Autodesk Fusion 360 part; units mm, degrees
note: some values were not read from the file. Chosen so that the rebuilt part matches the saved one: which bodies a step acts on; which face or edge a step refers to. Set by a fixed rule: which sketch regions a step uses.
(part 2 of 2)
  constraint coincident L37.end L318
  constraint collinear L368 L379
  constraint vertical L402
  constraint vertical L419
  constraint vertical L410
  constraint vertical L381
  constraint midpoint P2 L306
  constraint horizontal L424
  constraint vertical L427
  constraint vertical L414
  constraint horizontal L442
  constraint vertical L328
  constraint horizontal L440
  constraint horizontal L417
  constraint coincident L38.end L318
  constraint coincident L39.start L318
  constraint coincident L46.end L318
  constraint coincident L45.start L318
  constraint coincident L43.end L318
  constraint coincident L44.start L318
  constraint coincident L49.end L318
  constraint coincident L47.start L318
  constraint collinear L368 L424
  constraint collinear L424 L442
  constraint collinear L440 L442
  constraint collinear L417 L440
  constraint horizontal L421
  constraint vertical L413
  constraint vertical L395
  constraint horizontal L412
  constraint vertical L401
  constraint horizontal L429
  constraint horizontal L439
  constraint collinear L412 L421
  constraint collinear L412 L429
  constraint collinear L429 L439
  constraint horizontal L420
  constraint vertical L390
  constraint vertical L433
  constraint horizontal L358
  constraint vertical L378
  constraint collinear L358 L420
  constraint equal L368 L424
  constraint equal L424 L442
  constraint equal L440 L442
  constraint equal L417 L440
  constraint equal L417 L421
  constraint equal L412 L421
  constraint equal L412 L429
  constraint equal L429 L439
  constraint equal L420 L439
  constraint equal L358 L420
  constraint coincident L63.start L318
  constraint coincident L64.end L318
  constraint coincident L65.start L318
  constraint coincident L67.end L318
  constraint coincident L50.start L318
  constraint coincident L57.end L318
  constraint coincident L59.start L318
  constraint coincident L60.end L318
  constraint coincident L52.start L318
  constraint coincident L53.end L318
  constraint coincident L54.start L318
  constraint collinear L420 L439
  constraint collinear L417 L421
  constraint vertical L369
  constraint vertical L391
  constraint vertical L370
  constraint coincident L107.end L333
  constraint perpendicular L333 L356
  constraint coincident L80.start L333
  constraint perpendicular L333 L403
  constraint coincident L120.end L333
  constraint perpendicular L333 L343
  constraint collinear L303 L377
  constraint coincident L108.start L333
  constraint perpendicular L333 L371
  constraint perpendicular L330 L371
  constraint coincident L113.end L333
  constraint perpendicular L333 L351
  constraint coincident L119.start L333
  constraint perpendicular L333 L389
  constraint perpendicular L351 L375
  constraint coincident L86.end L333
  constraint perpendicular L333 L397
  constraint coincident L98.start L333
  constraint perpendicular L333 L380
  constraint perpendicular L351 L441
  constraint coincident L103.end L333
  constraint perpendicular L333 L382
  constraint coincident L128.start L333
  constraint perpendicular L333 L434
  constraint perpendicular L351 L405
  constraint coincident L130.end L333
  constraint perpendicular L333 L388
  constraint coincident L126.start L333
  constraint perpendicular L333 L357
  constraint perpendicular L351 L374
  constraint coincident L129.end L333
  constraint perpendicular L333 L372
  constraint equal L343 L371
  constraint equal L343 L389
  constraint equal L343 L380
  constraint equal L343 L434
  constraint equal L343 L357
  constraint equal L330 L377
  constraint equal L375 L377
  constraint equal L377 L441
  constraint equal L377 L405
  constraint equal L374 L377
  constraint perpendicular L360 L392
  constraint perpendicular L373 L376
  constraint perpendicular L376 L423
  constraint equal L384 L392
  constraint equal L363 L384
  constraint equal L384 L409
  constraint equal L354 L360
  constraint equal L354 L373
  constraint equal L354 L423
  constraint coincident L93.start L333
  constraint coincident L94.end L333
  constraint coincident L99.start L333
  constraint coincident L114.end L333
  constraint coincident L109.start L333
  constraint coincident L96.end L333
  constraint coincident L123.start L333
  constraint coincident L127.end L333
  constraint collinear L354 L377
  constraint coincident L118.end L333
  constraint coincident L112.start L333
  constraint coincident L88.end L333
  constraint coincident L72.start L333
  constraint coincident L85.end L333
  constraint coincident L71.start L333
  constraint coincident L121.end L333
  constraint coincident L74.start L333
  constraint collinear L307 L377
  constraint collinear L297 L307
  constraint collinear L297 L332
  constraint collinear L304 L332
  constraint collinear L302 L322
  constraint collinear L302 L338
  constraint collinear L327 L338
  constraint collinear L296 L311
  constraint equal L307 L377
  constraint equal L297 L307
  constraint equal L297 L332
  constraint equal L304 L332
  constraint equal L304 L322
  constraint equal L302 L322
  constraint equal L302 L338
  constraint equal L327 L338
  constraint equal L311 L327
  constraint equal L296 L311
  constraint coincident L115.start L333
  constraint coincident L70.end L333
  constraint coincident L111.start L333
  constraint coincident L101.end L333
  constraint coincident L84.start L333
  constraint coincident L91.end L333
  constraint coincident L100.start L333
  constraint coincident L83.end L333
  constraint coincident L97.start L333
  constraint coincident L82.end L333
  constraint coincident L110.start L333
  constraint collinear L311 L327
  constraint collinear L304 L322
  constraint horizontal L333
  constraint coincident L76.start L347
  constraint coincident L7.start L333
  constraint coincident L8.start L333
  constraint coincident L76.end L341
  constraint coincident L9.start L333
  constraint coincident L14.start L333
  constraint coincident L131.end L333
  constraint perpendicular L331 L333
  constraint collinear L331 L437
  constraint collinear L356 L400
  constraint vertical L384
  constraint vertical L376
  constraint vertical L416
  constraint vertical L435
  constraint vertical L301
  constraint vertical L323
  constraint vertical L300
  constraint vertical L312
  constraint vertical L308
  constraint vertical L324
  constraint vertical L317
  constraint vertical L299
  constraint vertical L314
  constraint vertical L310
  constraint vertical L316
  constraint coincident L102.end L333
  constraint collinear L301 L427
  constraint perpendicular L349 L393
  constraint perpendicular L365 L396
  constraint perpendicular L365 L431
  constraint vertical L393
  constraint vertical L387
  constraint vertical L418
  constraint vertical L428
  constraint coincident L136.end L318
  constraint coincident L139.start L318
  constraint coincident L140.end L318
  constraint coincident L135.start L318
  constraint coincident L137.end L318
  constraint coincident L132.start L318
  constraint coincident L58.end L318
  constraint coincident L143.start L318
  constraint perpendicular L318 L415
  constraint perpendicular L415 L432
  constraint coincident L145.end L318
  constraint perpendicular L318 L364
  constraint collinear L379 L432
  constraint equal L379 L432
  constraint equal L364 L428
  constraint equal L426 L428
  constraint equal L365 L426
  constraint equal L431 L432
  constraint equal L396 L431
  constraint vertical L359
  constraint perpendicular L336 L379
  measures "d1" distance of L0.end L1.end
  measures "d2" distance of L1.end L2.end
  measures "d4" distance of L3 L9
  measures "d5" distance of L0 L6
  measures "d7" distance of L7 L8
  measures "d8" distance of L6 L11
  measures "d11" distance of L9 L14
  measures "d12" distance of L0 L16
  measures "d13" distance of L15.end L16.end
  measures "d14" distance of L8 L17
  measures "d15" distance of L6 L18
  measures "d17" distance of L19 L20
  measures "d18" distance of L20.end L21.end
  measures "d19" distance of L22 L23
  measures "d24" distance of L27.end L26.start
  measures "d25" distance of L26 L34
  measures "d26" distance of L31 L35
  measures "d27" distance of L28 L32
  measures "d33" distance of L14 L19
  measures "d37" distance of L44 L49
  measures "d38" distance of L43 L45
  measures "d39" distance of L39 L46
  measures "d40" distance of L57 L59
  measures "d41" distance of L52 L60
  measures "d42" distance of L53 L54
  measures "d45" distance of L64 L65
  measures "d46" distance of L17 L38
  measures "d47" distance of L47 L58
  measures "d48" distance of L50 L67
  measures "d50" distance of L69 L76
  measures "d51" distance of L80 L107
  measures "d52" distance of L80.end L106.end
  measures "d53" distance of L108 L120
  measures "d54" distance of L113 L119
  measures "d55" distance of L86 L98
  measures "d56" distance of L103 L128
  measures "d57" distance of L126 L130
  measures "d58" distance of L78.end L78.start
  measures "d59" distance of L94 L99
  measures "d60" distance of L109 L114
  measures "d61" distance of L96 L123
  measures "d64" distance of L93 L129
  measures "d68" distance of L71 L121
  measures "d69" distance of L72 L85
  measures "d70" distance of L88 L112
  measures "d71" distance of L91 L100
  measures "d72" distance of L83 L97
  measures "d73" distance of L82 L110
  measures "d76" distance of L70 L111
  measures "d77" distance of L74 L102
  measures "d78" distance of L84 L101
  measures "d81" distance of L135 L137
  measures "d82" distance of L139 L140
  measures "d99" distance of L2 L76
  measures "d100" distance of L10 L76
  measures "d102" distance of L14 P2
  measures "d103" distance of L8 L14
  measures "d104" distance of L27 L143
  measures "d105" distance of L136 L145
  measures "d106" distance of L25 L132
  measures "d128" diameter of A0
  measures "d129" horizontal distance of L15.end A0.centre
  measures "d130" vertical distance of L15.end A0.centre
  measures "d131" diameter of A1
  measures "d132" horizontal distance of L16.end A1.centre
  measures "d139" distance of L0.end L1.end
  measures "d140" distance of L1.end L2.end
  measures "d141" distance of L193 L198
  measures "d142" distance of L170 L191
  measures "d143" distance of L187 L194
  measures "d144" distance of L170 L274
  measures "d145" distance of L186 L198
  measures "d146" distance of L158 L191
  measures "d147" distance of L15.end L16.end
  measures "d148" distance of L187 L289
  measures "d149" distance of L170 L202
  measures "d150" distance of L181 L252
  measures "d151" distance of L20.end L21.end
  measures "d152" distance of L235 L246
  measures "d153" distance of L26.start L27.end
  measures "d154" distance of L271 L282
  measures "d155" distance of L262 L288
  measures "d156" distance of L233 L237
  measures "d157" distance of L186 L252
  measures "d158" distance of L243 L260
  measures "d159" distance of L180 L204
  measures "d160" distance of L251 L266
  measures "d161" distance of L213 L222
  measures "d162" distance of L207 L253
  measures "d163" distance of L247 L259
  measures "d164" distance of L250 L285
  measures "d165" distance of L279 L289
  measures "d166" distance of L221 L265
  measures "d167" distance of L242 L295
  measures "d168" distance of L155 L185
  measures "d169" distance of L208 L255
  measures "d170" distance of L106.end L80.end
  measures "d171" distance of L195 L223
  measures "d172" distance of L203 L241
  measures "d173" distance of L232 L249
  measures "d174" distance of L234 L286
  measures "d175" distance of L209 L240
  measures "d176" distance of L78.end L78.start
  measures "d177" distance of L236 L244
  measures "d178" distance of L215 L228
  measures "d179" distance of L261 L268
  measures "d180" distance of L214 L224
  measures "d181" distance of L164 L197
  measures "d182" distance of L152 L189
  measures "d183" distance of L172 L175
  measures "d184" distance of L151 L196
  measures "d185" distance of L169 L171
  measures "d186" distance of L157 L176
  measures "d187" distance of L150 L166
  measures "d188" distance of L160 L161
  measures "d189" distance of L162 L167
  measures "d190" distance of L217 L239
  measures "d191" distance of L270 L278
  measures "d192" distance of L165 L185
  measures "d193" distance of L173 L185
  measures "d194" distance of P2 L186
  measures "d195" distance of L186 L187
  measures "d196" distance of L254 L267
  measures "d197" distance of L216 L280
  measures "d198" distance of L205 L245
  measures "d199" diameter of A2
  measures "d200" horizontal distance of L15.end A0.centre
  measures "d201" vertical distance of L15.end A0.centre
  measures "d202" diameter of A3
  measures "d203" horizontal distance of L16.end A1.centre
  measures "d204" distance of L0.end L1.end
  measures "d205" distance of L1.end L2.end
  measures "d206" distance of L341 L346
  measures "d207" distance of L318 L339
  measures "d208" distance of L335 L342
  measures "d209" distance of L318 L422
  measures "d210" distance of L334 L346
  measures "d211" distance of L306 L339
  measures "d212" distance of L15.end L16.end
  measures "d213" distance of L335 L437
  measures "d214" distance of L318 L350
  measures "d215" distance of L329 L400
  measures "d216" distance of L20.end L21.end
  measures "d217" distance of L383 L394
  measures "d218" distance of L26.start L27.end
  measures "d219" distance of L419 L430
  measures "d220" distance of L410 L436
  measures "d221" distance of L381 L385
  measures "d222" distance of L334 L400
  measures "d223" distance of L391 L408
  measures "d224" distance of L328 L352
  measures "d225" distance of L399 L414
  measures "d226" distance of L361 L370
  measures "d227" distance of L355 L401
  measures "d228" distance of L395 L407
  measures "d229" distance of L398 L433
  measures "d230" distance of L427 L437
  measures "d231" distance of L369 L413
  measures "d232" distance of L390 L443
  measures "d233" distance of L303 L333
  measures "d234" distance of L356 L403
  measures "d235" distance of L106.end L80.end
  measures "d236" distance of L343 L371
  measures "d237" distance of L351 L389
  measures "d238" distance of L380 L397
  measures "d239" distance of L382 L434
  measures "d240" distance of L357 L388
  measures "d241" distance of L78.end L78.start
  measures "d242" distance of L384 L392
  measures "d243" distance of L363 L376
  measures "d244" distance of L409 L416
  measures "d245" distance of L362 L372
  measures "d246" distance of L312 L345
  measures "d247" distance of L300 L337
  measures "d248" distance of L320 L323
  measures "d249" distance of L299 L344
  measures "d250" distance of L317 L319
  measures "d251" distance of L305 L324
  measures "d252" distance of L298 L314
  measures "d253" distance of L308 L309
  measures "d254" distance of L310 L315
  measures "d255" distance of L365 L387
  measures "d256" distance of L418 L426
  measures "d257" distance of L313 L333
  measures "d258" distance of L321 L333
  measures "d259" distance of P2 L334
  measures "d260" distance of L334 L335
  measures "d261" distance of L402 L415
  measures "d262" distance of L364 L428
  measures "d263" distance of L353 L393
  measures "d264" diameter of A4
  measures "d265" horizontal distance of L15.end A0.centre
  measures "d266" vertical distance of L15.end A0.centre
  measures "d267" diameter of A5
  measures "d268" horizontal distance of L16.end A1.centre
extrude "Extrude1" add sketch "Sketch1" along normal blind 438.15 from surface at -57.15 contours L0 L3 L6 L17 L170 L191 L193 L289 L318 L339 L341 L437 | L0 L1 L6 L15 L170 L191 L199 L256 L318 L339 L347 L404 | L1 L2 L3 L76 L165 L185 L193 L199 L313 L333 L341 L347 makes body 1 at (-162.9833, -273.05, 88.9) makes body 2 at (239.1833, 254, 234.95) makes body 3 at (416.9833, -254, 88.9) in component "Large Box"
extrude "Extrude2" add sketch "Sketch1" along normal up to surface (381 mm away) separate body contours L3 L6 L9 L11 L170 L193 L198 L274 L318 L341 L346 L422 | L3 L9 L10 L76 L173 L185 L193 L198 L321 L333 L341 L346 | L1 L6 L7 L13 L170 L194 L199 L258 L318 L342 L347 L406 | L1 L7 L12 L76 L185 L194 L199 L238 L333 L342 L347 L386 makes body 4 at (-717.55, -241.3, 127) makes body 5 at (692.15, -254, 127) makes body 6 at (-692.15, 215.9, 127) makes body 7 at (717.55, 241.3, 127) in component "Large Box"
extrude "Extrude3" add sketch "Sketch1" along normal up to surface (381 mm away) separate body contours L6 L9 L14 L76 L170 L185 L186 L198 L318 L333 L334 L346 | L6 L7 L8 L76 L170 L185 L187 L194 L318 L333 L335 L342 makes body 8 at (-679.45, 84.6667, 127) makes body 9 at (679.45, 84.6667, 127) in component "Large Box"
extrude "Extrude4" add sketch "Sketch1" along normal up to surface (361.95 mm away) separate body contours L6 L15 L18 L19 L170 L202 L252 L256 L318 L350 L400 L404 | L6 L38 L39 L41 L170 L266 L276 L279 L318 L414 L424 L427 | L6 L63 L64 L66 L170 L210 L230 L250 L318 L358 L378 L398 | L6 L20 L21 L22 L170 L181 L220 L235 L318 L329 L368 L383 | L6 L45 L46 L48 L170 L180 L251 L294 L318 L328 L399 L442 | L70 L75 L76 L115 L148 L150 L168 L185 L296 L298 L316 L333 | L6 L62 L65 L67 L170 L242 L272 L285 L318 L390 L420 L433 | L6 L30 L32 L37 L170 L211 L233 L263 L318 L359 L381 L411 | L6 L23 L24 L25 L170 L205 L218 L246 L318 L353 L366 L394 | L6 L42 L43 L44 L170 L204 L260 L292 L318 L352 L408 L440 | L73 L76 L101 L111 L163 L166 L167 L185 L311 L314 L315 L333 | L76 L105 L123 L127 L185 L261 L275 L287 L333 L409 L423 L435 | L6 L50 L56 L57 L170 L213 L291 L295 L318 L361 L439 L443 | L6 L28 L29 L35 L170 L237 L262 L277 L318 L385 L410 L425 | L6 L132 L134 L137 L170 L201 L217 L245 L318 L349 L365 L393 | L6 L40 L47 L49 L170 L221 L243 L269 L318 L369 L391 L417 | L76 L77 L84 L91 L162 L179 L185 L196 L310 L327 L333 L344 | L76 L89 L96 L109 L185 L215 L225 L268 L333 L363 L373 L416 | L6 L59 L60 L61 L170 L207 L222 L281 L318 L355 L370 L429 | L6 L31 L34 L36 L170 L271 L288 L290 L318 L419 L436 L438 | L6 L135 L138 L140 L170 L239 L248 L278 L318 L387 L396 L426 | L6 L51 L54 L58 L170 L247 L265 L273 L318 L395 L413 L421 | L76 L83 L95 L100 L151 L171 L185 L190 L299 L319 L333 L338 | L76 L99 L114 L117 L185 L212 L228 L244 L333 L360 L376 L392 | L74 L76 L87 L121 L156 L160 L185 L197 L304 L308 L333 L345 | L6 L52 L53 L55 L170 L253 L259 L264 L318 L401 L407 L412 | L6 L26 L27 L33 L170 L231 L254 L282 L318 L379 L402 L430 | L6 L133 L136 L139 L170 L270 L280 L283 L318 L418 L428 L431 | L76 L102 L110 L124 L161 L174 L176 L185 L309 L322 L324 L333 | L76 L82 L90 L97 L154 L157 L169 L185 L302 L305 L317 L333 | L76 L78 L93 L94 L185 L206 L214 L236 L333 L354 L362 L384 | L6 L143 L144 L145 L170 L216 L267 L284 L318 L364 L415 L432 | L71 L76 L85 L122 L164 L184 L185 L189 L312 L332 L333 L337 | L76 L125 L126 L129 L185 L209 L224 L226 L333 L357 L372 L374 | L72 L76 L88 L104 L149 L152 L172 L185 L297 L300 L320 L333 | L76 L92 L128 L130 L185 L240 L257 L286 L333 L388 L405 L434 | L76 L79 L112 L118 L153 L159 L175 L185 L301 L307 L323 L333 | L68 L76 L98 L103 L185 L232 L234 L293 L333 L380 L382 L441 | L69 L76 L107 L131 L155 L183 L185 L208 L303 L331 L333 L356 | L76 L81 L86 L119 L185 L227 L241 L249 L333 L375 L389 L397 | L76 L80 L106 L120 L185 L195 L229 L255 L333 L343 L377 L403 | L76 L108 L113 L116 L182 L185 L203 L223 L330 L333 L351 L371 makes body 10 at (374.65, 234.95, 120.65) makes body 11 at (603.2275, 234.95, 120.65) makes body 12 at (-647.7, 241.3, 120.65) makes body 13 at (527.0275, 234.95, 241.3) makes body 14 at (634.9775, -254, 120.65) makes body 15 at (488.9275, -234.95, 120.65) makes body 16 at (330.2, -254, 241.3) makes body 17 at (-342.9, -241.3, 120.65) makes body 18 at (-476.25, -241.3, 120.65) makes body 19 at (-628.65, -247.65, 120.65) makes body 20 at (-381, 241.3, 120.65) makes body 21 at (-514.35, 247.65, 120.65) makes body 22 at (-476.25, 247.65, 120.65) makes body 23 at (-342.9, 241.3, 120.65) makes body 24 at (-590.55, -247.65, 120.65) makes body 25 at (-450.85, -254, 120.65) makes body 26 at (-304.8, -241.3, 120.65) makes body 27 at (374.65, -234.95, 120.65) makes body 28 at (527.0275, -234.95, 120.65) makes body 29 at (634.9775, 254, 120.65) makes body 30 at (488.9275, 234.95, 241.3) makes body 31 at (336.55, 234.95, 120.65) makes body 32 at (406.4, 254, 120.65) makes body 33 at (558.7775, 254, 120.65) makes body 34 at (603.2275, -234.95, 120.65) makes body 35 at (444.4775, -254, 120.65) makes body 36 at (292.1, -254, 120.65) makes body 37 at (-381, -241.3, 120.65) makes body 38 at (-533.4, -241.3, 241.3) makes body 39 at (88.9, 234.95, 241.3) makes body 40 at (-419.1, 241.3, 120.65) makes body 41 at (-571.5, 241.3, 120.65) makes body 42 at (-609.6, 241.3, 120.65) makes body 43 at (-438.15, 247.65, 120.65) makes body 44 at (-304.8, 241.3, 120.65) makes body 45 at (-552.45, -247.65, 241.3) makes body 46 at (-419.1, -241.3, 120.65) makes body 47 at (-12.7, -234.95, 120.65) makes body 48 at (406.4, -254, 120.65) makes body 49 at (565.1275, -234.95, 120.65) makes body 50 at (450.8275, 234.95, 120.65) makes body 51 at (298.45, 234.95, 120.65) in component "Large Box"
extrude "Extrude5" add sketch "Sketch1" against normal blind 19.05 separate body contours L3 L6 L9 L11 L170 L193 L198 L274 L318 L341 L346 L422 | L6 L15 L16 L17 L18 L19 L20 L21 L22 L23 L24 L25 L38 L39 L40 L41 L42 L43 L44 L45 L46 L48 L49 L68 L69 L71 L72 L76 L79 L80 L81 L85 L86 L87 L88 L92 L98 L103 L104 L106 L107 L108 L112 L113 L116 L118 L119 L120 L121 L122 L125 L126 L128 L130 L131 L132 L133 L134 L135 L136 L137 L138 L139 L140 L141 L144 L145 L147 L149 L152 L153 L155 L156 L158 L159 L164 L170 L172 L175 L180 L181 L182 L183 L184 L185 L189 L192 L195 L197 L201 L202 L203 L204 L205 L208 L209 L216 L217 L218 L219 L220 L223 L226 L227 L229 L232 L234 L235 L239 L240 L241 L243 L245 L246 L248 L249 L251 L252 L255 L256 L257 L260 L266 L269 L270 L276 L278 L279 L280 L283 L284 L286 L289 L292 L293 L294 L297 L300 L301 L303 L304 L306 L307 L312 L318 L320 L323 L328 L329 L330 L331 L332 L333 L337 L340 L343 L345 L349 L350 L351 L352 L353 L356 L357 L364 L365 L366 L367 L368 L371 L374 L375 L377 L380 L382 L383 L387 L388 L389 L391 L393 L394 L396 L397 L399 L400 L403 L404 L405 L408 L414 L417 L418 L424 L426 L427 L428 L431 L432 L434 L437 L440 L441 L442 | L3 L9 L10 L11 L173 L193 L198 L274 L321 L341 L346 L422 | L6 L9 L14 L76 L170 L185 L186 L198 L318 L333 L334 L346 | L6 L15 L18 L19 L170 L202 L252 L256 L318 L350 L400 L404 | L6 L38 L39 L41 L170 L266 L276 L279 L318 L414 L424 L427 | L3 L9 L10 L76 L173 L185 L193 L198 L321 L333 L341 L346 | L6 L14 L50 L51 L52 L53 L54 L55 L56 L57 L59 L60 L61 L62 L63 L64 L65 L66 L67 L70 L73 L75 L76 L77 L82 L83 L84 L90 L91 L95 L97 L100 L101 L110 L111 L115 L124 L142 L148 L150 L151 L154 L157 L162 L163 L166 L167 L168 L169 L170 L171 L174 L176 L179 L185 L186 L190 L196 L200 L207 L210 L213 L222 L230 L242 L247 L250 L253 L259 L264 L272 L273 L281 L285 L291 L295 L296 L298 L299 L302 L305 L310 L311 L314 L315 L316 L317 L318 L319 L322 L324 L327 L333 L334 L338 L344 L348 L355 L358 L361 L370 L378 L390 L395 L398 L401 L407 L412 L420 L421 L429 L433 L439 L443 | L1 L6 L7 L13 L170 L194 L199 L258 L318 L342 L347 L406 | L6 L63 L64 L66 L170 L210 L230 L250 L318 L358 L378 L398 | L1 L7 L12 L13 L194 L199 L238 L258 L342 L347 L386 L406 | L6 L7 L8 L76 L170 L185 L187 L194 L318 L333 L335 L342 | L6 L20 L21 L22 L170 L181 L220 L235 L318 L329 L368 L383 | L6 L45 L46 L48 L170 L180 L251 L294 L318 L328 L399 L442 | L70 L75 L76 L115 L148 L150 L168 L185 L296 L298 L316 L333 | L1 L7 L12 L76 L185 L194 L199 L238 L333 L342 L347 L386 | L6 L8 L26 L28 L29 L30 L31 L32 L33 L34 L35 L36 L37 L76 L78 L89 L94 L96 L99 L105 L109 L114 L117 L123 L127 L146 L170 L185 L187 L188 L206 L211 L212 L215 L225 L228 L231 L233 L236 L237 L244 L261 L262 L263 L268 L271 L275 L277 L282 L287 L288 L290 L318 L333 L335 L336 L354 L359 L360 L363 L373 L376 L379 L381 L384 L385 L392 L409 L410 L411 L416 L419 L423 L425 L430 L435 L436 L438 | L6 L62 L65 L67 L170 L242 L272 L285 L318 L390 L420 L433 | L6 L30 L32 L37 L170 L211 L233 L263 L318 L359 L381 L411 | L6 L23 L24 L25 L170 L205 L218 L246 L318 L353 L366 L394 | L6 L42 L43 L44 L170 L204 L260 L292 L318 L352 L408 L440 | L73 L76 L101 L111 L163 L166 L167 L185 L311 L314 L315 L333 | L76 L105 L123 L127 L185 L261 L275 L287 L333 L409 L423 L435 | L6 L50 L56 L57 L170 L213 L291 L295 L318 L361 L439 L443 | L6 L28 L29 L35 L170 L237 L262 L277 L318 L385 L410 L425 | L6 L132 L134 L137 L170 L201 L217 L245 L318 L349 L365 L393 | L6 L40 L47 L49 L170 L221 L243 L269 L318 L369 L391 L417 | L76 L77 L84 L91 L162 L179 L185 L196 L310 L327 L333 L344 | L76 L89 L96 L109 L185 L215 L225 L268 L333 L363 L373 L416 | L6 L47 L58 L74 L76 L102 L141 L142 L160 L161 L170 L185 L192 L200 L221 L265 L308 L309 L318 L333 L340 L348 L369 L413 | L6 L59 L60 L61 L170 L207 L222 L281 L318 L355 L370 L429 | L6 L31 L34 L36 L170 L271 L288 L290 L318 L419 L436 L438 | L6 L135 L138 L140 L170 L239 L248 L278 L318 L387 L396 L426 | L6 L51 L54 L58 L170 L247 L265 L273 L318 L395 L413 L421 | L76 L83 L95 L100 L151 L171 L185 L190 L299 L319 L333 L338 | L76 L99 L114 L117 L185 L212 L228 L244 L333 L360 L376 L392 | L74 L76 L87 L121 L156 L160 L185 L197 L304 L308 L333 L345 | L6 L52 L53 L55 L170 L253 L259 L264 L318 L401 L407 L412 | L6 L26 L27 L33 L170 L231 L254 L282 L318 L379 L402 L430 | L6 L133 L136 L139 L170 L270 L280 L283 L318 L418 L428 L431 | L76 L102 L110 L124 L161 L174 L176 L185 L309 L322 L324 L333 | L76 L82 L90 L97 L154 L157 L169 L185 L302 L305 L317 L333 | L6 L27 L76 L93 L129 L143 L146 L147 L170 L185 L188 L214 L219 L224 L254 L267 L318 L333 L336 L362 L367 L372 L402 L415 | L76 L78 L93 L94 L185 L206 L214 L236 L333 L354 L362 L384 | L6 L143 L144 L145 L170 L216 L267 L284 L318 L364 L415 L432 | L71 L76 L85 L122 L164 L184 L185 L189 L312 L332 L333 L337 | L76 L125 L126 L129 L185 L209 L224 L226 L333 L357 L372 L374 | L72 L76 L88 L104 L149 L152 L172 L185 L297 L300 L320 L333 | L76 L92 L128 L130 L185 L240 L257 L286 L333 L388 L405 L434 | L76 L79 L112 L118 L153 L159 L175 L185 L301 L307 L323 L333 | L68 L76 L98 L103 L185 L232 L234 L293 L333 L380 L382 L441 | L69 L76 L107 L131 L155 L183 L185 L208 L303 L331 L333 L356 | L76 L81 L86 L119 L185 L227 L241 L249 L333 L375 L389 L397 | L76 L80 L106 L120 L185 L195 L229 L255 L333 L343 L377 L403 | L76 L108 L113 L116 L182 L185 L203 L223 L330 L333 L351 L371 | A0 A2 A4 | A1 A3 A5 makes body 52 in component "Large Box"
sketch "Sketch2" plane through (0, 0, 0) normal (0, 0, 1) x (1, 0, 0) in component "Large Box"
  line L0 (-660.4, 254) -> (660.4, 254)
  line L1 (660.4, 254) -> (660.4, -254)
  line L2 (660.4, -254) -> (266.7, -254)
  line L3 (266.7, -254) -> (266.7, -82.55)
  line L4 (266.7, -82.55) -> (114.3, -82.55)
  line L5 (114.3, -82.55) -> (114.3, -254)
  line L6 (114.3, -254) -> (-660.4, -254)
  line L7 (-660.4, -254) -> (-660.4, 254)
  line L8 (114.3, -82.55) -> (-25.4, -82.55)
  line L9 (-25.4, -82.55) -> (-25.4, -254)
  line L10 (266.7, -82.55) -> (406.4, -82.55)
  line L11 (406.4, -82.55) -> (406.4, -254)
  line L12 (406.4, -82.55) -> (406.4, 57.15)
  line L13 (406.4, 57.15) -> (-25.4, 57.15)
  line L14 (-25.4, 57.15) -> (-25.4, -82.55)
  line L15 (-660.4, 254) -> (-717.55, 254)
  line L16 (-717.55, 254) -> (-717.55, 215.9)
  line L17 (-717.55, 215.9) -> (717.55, 215.9)
  line L18 (717.55, 215.9) -> (717.55, 254)
  line L19 (717.55, 254) -> (660.4, 254)
  line L20 (-660.4, -254) -> (-717.55, -254)
  line L21 (-717.55, -254) -> (-717.55, -215.9)
  line L22 (-717.55, -215.9) -> (-25.4, -215.9)
  line L23 (660.4, -254) -> (717.55, -254)
  line L24 (717.55, -254) -> (717.55, -215.9)
  line L25 (717.55, -215.9) -> (406.4, -215.9)
  line L26 (-25.4, -215.9) -> (114.3, -215.9)
  line L27 (406.4, -215.9) -> (266.7, -215.9)
  point P0 (-660.4, 254)
  point P1 (-660.4, -254)
  point P2 (114.3, -82.55)
  point P3 (266.7, -82.55)
  point P4 (660.4, 254)
  point P5 (660.4, -254)
  point P6 (-717.55, -254)
  point P7 (717.55, -254)
  point P8 (717.55, 254)
  point P9 (-717.55, 254)
  point P10 (-717.55, 273.05)
  point P11 (717.55, 273.05)
  point P12 (717.55, -273.05)
  point P13 (-717.55, -273.05)
  dimension "d108" = 139.7
  dimension "d109" = 139.7
  dimension "d110" = 139.7
  dimension "d111" = 38.1
  dimension "d112" = 38.1
  constraint coincident P0 L0.start
  constraint coincident P4 L0.end
  constraint coincident P5 L1.end
  constraint perpendicular L1 L2
  constraint coincident P3 L3.end
  constraint coincident P2 L4.end
  constraint coincident P1 L6.end
  constraint vertical L5
  constraint horizontal L6
  constraint vertical L3
  constraint perpendicular L5 L8
  constraint coincident L6 L9.end
  constraint perpendicular L6 L9
  constraint perpendicular L3 L10
  constraint coincident L2 L11.end
  constraint perpendicular L2 L11
  constraint perpendicular L10 L12
  constraint perpendicular L11 L13
  constraint vertical L14
  constraint coincident P9 L15.end
  constraint perpendicular L0 L16
  constraint perpendicular L7 L17
  constraint coincident P8 L18.end
  constraint coincident P6 L20.end
  constraint perpendicular L20 L21
  constraint coincident L9 L22.end
  constraint perpendicular L9 L22
  constraint coincident P7 L23.end
  constraint perpendicular L2 L24
  constraint coincident L11 L25.end
  constraint collinear L22 L25
  constraint vertical L18
  constraint coincident L5 L26.end
  constraint perpendicular L5 L26
  constraint coincident L3 L27.end
  constraint perpendicular L3 L27
  measures "d108" distance of L5 L9
  measures "d109" distance of L3 L11
  measures "d110" distance of L4 L13
  measures "d111" distance of L6 L22
  measures "d112" distance of L0 L17
extrude "Extrude7" add sketch "Sketch2" against normal up to surface (38.1 mm away) from surface at -19.05 separate body contours L0 L1 L7 L17 | L7 L15 L16 L17 | L1 L17 L18 L19 | L6 L7 L9 L22 | L7 L20 L21 L22 | L1 L23 L24 L25 | L1 L2 L11 L25 makes body 53 at (-239.1833, 254, -31.75) makes body 54 at (-256.1167, -254, -44.45) makes body 55 at (613.8333, -254, -31.75) in component "Large Box"
extrude "Extrude6" add sketch "Sketch2" along normal blind 19.05 from surface at 762 separate body contours L0 L1 L7 L17 | L1 L7 L9 L11 L12 L13 L14 L17 L22 L25 | L6 L7 L9 L22 | L1 L2 L11 L25 | L5 L6 L9 L26 | L5 L8 L9 L26 | L3 L10 L11 L27 | L2 L3 L11 L27 | L4 L8 L10 L12 L13 L14 makes body 56 in component "Large Box"
extrude "Extrude1'" add sketch "Sketch1" along normal blind 355.6 separate body contours L6 L47 L58 L74 L76 L102 L141 L142 L160 L161 L170 L185 L192 L200 L221 L265 L308 L309 L318 L333 L340 L348 L369 L413 | L6 L27 L76 L93 L129 L143 L146 L147 L170 L185 L188 L214 L219 L224 L254 L267 L318 L333 L336 L362 L367 L372 L402 L415 makes body 57 at (-514.35, 84.6667, 118.5333) makes body 58 at (419.1, -84.6667, 237.0667) in component "Moving Walls"
extrude "Extrude1''" add sketch "Sketch2" against normal up to surface (38.1 mm away) from surface at -19.05 separate body contours L5 L6 L9 L26 | L5 L8 L9 L26 | L3 L10 L11 L27 | L2 L3 L11 L27 makes body 59 at (359.8333, -139.7, -19.05) makes body 60 at (21.1667, -139.7, -19.05) in component "Sacrificial Sides"
extrude "Extrude2'" add sketch "Sketch2" against normal up to surface (38.1 mm away) from surface at -19.05 separate body contours L4 L8 L10 L12 L13 L14 makes body 61 in component "Sacrificial Sides"
extrude "Extrude3'" add sketch "Sketch2" along normal blind 38.1 from surface at 781.05 separate body contours L5 L6 L9 L26 | L5 L8 L9 L26 | L3 L10 L11 L27 | L2 L3 L11 L27 makes body 62 at (21.1667, -139.7, 781.05) makes body 63 at (359.8333, -139.7, 781.05) in component "Sacrificial Sides"
extrude "Extrude4'" add sketch "Sketch2" along normal up to surface (38.1 mm away) from surface at 781.05 separate body contours L4 L8 L10 L12 L13 L14 makes body 64 in component "Sacrificial Sides"
extrude "Extrude1'''" add sketch "Sketch1" against normal blind 50.8 from surface at 762 separate body contours A0 A2 A4 | A1 A3 A5 makes body 65 at (92.9638, -54.6667, 728.1333) makes body 66 at (288.7746, -53.7407, 728.1333) in component "Pegs"
extrude "Extrude2''" add sketch "Sketch1" along normal blind 50.8 separate body contours A0 A2 A4 | A1 A3 A5 makes body 67 at (92.9638, -54.6667, 33.8667) makes body 68 at (288.7746, -53.7407, 33.8667) in component "Pegs"
move_body "Move1" bodies 56 to x (1, 0, 0) y (0, 1, 0) z (0, 0, 1) at (0, 0, -400.05) in component "Large Box"
move_body "Move1'" bodies 62 63 64 to x (1, 0, 0) y (0, 1, 0) z (0, 0, 1) at (0, 0, -400.05) in component "Sacrificial Sides"
move_body "Move1''" bodies 65 66 to x (1, 0, 0) y (0, 1, 0) z (0, 0, 1) at (0, 0, -400.05) in component "Pegs"
sketch "Sketch1 (2)" plane through (0, 0, 0) normal (0, 0, 1) x (1, 0, 0) in component "Saddle"
  line L0 (-76.2, 15.875) -> (76.2, 15.875)
  line L1 (-406.4, 155.575) -> (406.4, 155.575)
  line L2 (-406.4, -136.525) -> (-76.2, -136.525)
  line L3 (406.4, -155.575) -> (-406.4, 155.575) construction
  line L4 (-406.4, -155.575) -> (406.4, 155.575) construction
  circle A0 centre (-101.6, 41.275) radius 4.7625
  line L5 (-76.2, -98.425) -> (-406.4, -98.425)
  line L6 (-76.2, -155.575) -> (-76.2, 15.875)
  line L7 (76.2, 15.875) -> (76.2, -155.575)
  line L8 (-406.4, 155.575) -> (-406.4, -155.575)
  line L9 (406.4, 155.575) -> (406.4, -155.575)
  line L10 (76.2, -98.425) -> (406.4, -98.425)
  line L11 (76.2, -136.525) -> (406.4, -136.525)
  line L12 (-215.9, -98.425) -> (-215.9, 155.575)
  line L13 (-76.2, 155.575) -> (-76.2, 15.875)
  line L14 (76.2, 15.875) -> (76.2, 155.575)
  line L15 (215.9, 155.575) -> (215.9, -98.425)
  circle A1 centre (101.6, 41.275) radius 4.7625
  line L16 (406.4, -155.575) -> (76.2, -155.575)
  line L17 (-76.2, -155.575) -> (-406.4, -155.575)
  point P0 (0, 15.875)
  dimension "d270" = 812.8
  dimension "d277" = 152.4
  dimension "d279" = 38.1
  dimension "d329" = 9.525
  dimension "d330" = 25.4
  dimension "d331" = 25.4
  dimension "d338" = 139.7
  dimension "d340" = 9.525
  dimension "d341" = 25.4
  dimension "d342" = 152.4
  dimension "d345" = 139.7
  dimension "d346" = 19.05
  dimension "d347" = 139.7
  dimension "d348" = 292.1
  constraint horizontal L16
  constraint coincident origin L3
  constraint coincident origin L4
  constraint coincident L6.start L16
  constraint perpendicular L6 L16
  constraint perpendicular L0 L6
  constraint perpendicular L7 L16
  constraint coincident L5.start L6
  constraint perpendicular L5 L6
  constraint midpoint P0 L0
  constraint horizontal L1
  constraint perpendicular L8 L16
  constraint perpendicular L9 L16
  constraint coincident L7 L10.start
  constraint perpendicular L7 L10
  constraint collinear L5 L10
  constraint coincident L5.end L8
  constraint coincident L2.start L8
  constraint coincident L2.end L6
  constraint coincident L9 L10.end
  constraint vertical origin P0
  constraint coincident L7 L11.start
  constraint coincident L9 L11.end
  constraint perpendicular L9 L11
  constraint collinear L2 L11
  constraint coincident L5 L12.start
  constraint perpendicular L5 L12
  constraint perpendicular L0 L14
  constraint coincident L10 L15.end
  constraint perpendicular L10 L15
  constraint vertical L13
  constraint horizontal A0.centre A1.centre
  constraint horizontal L17
  constraint coincident L1 L12.end
  constraint coincident L1 L13.start
  constraint coincident L1 L14.end
  constraint coincident L1 L15.start
  measures "d270" distance of L1.start L1.end
  measures "d277" distance of L0.start L0.end
  measures "d279" distance of L2 L5
  measures "d329" diameter of A0
  measures "d330" horizontal distance of L0.start A0.centre
  measures "d331" vertical distance of L0.start A0.centre
  measures "d338" distance of L12.end L13.start
  measures "d340" diameter of A1
  measures "d341" horizontal distance of L0.end A1.centre
  measures "d342" distance of L0 L2
  measures "d345" distance of L0 L1
  measures "d346" distance of L2 L17
  measures "d347" distance of L14 L15
  measures "d348" distance of L1 L2
extrude "Extrude1''''" add sketch "Sketch1 (2)" against normal blind 19.05 from surface at -368.3 separate body contours L0 L1 L13 L14 | L1 L5 L6 L12 L13 | L1 L7 L10 L14 L15 | L2 L5 L6 L8 | L7 L9 L10 L11 | L1 L5 L8 L12 | L1 L9 L10 L15 | A0 | A1 makes body 69 in component "Saddle"
extrude "Extrude2'''" add sketch "Sketch1 (2)" along normal blind 19.05 separate body contours L0 L1 L13 L14 | L1 L5 L6 L12 L13 | L1 L7 L10 L14 L15 | L2 L5 L6 L8 | L7 L9 L10 L11 | L1 L5 L8 L12 | L1 L9 L10 L15 | A0 | A1 makes body 70 in component "Saddle"
extrude "Extrude3''" add sketch "Sketch1 (2)" against normal up to surface (482.6 mm away) from surface at 57.15 separate body contours L2 L6 L8 L17 | L7 L9 L11 L16 makes body 71 at (-186.2667, -136.525, -264.5833) makes body 72 at (296.3333, -155.575, -103.7167) in component "Saddle"
extrude "Extrude1'''''" add sketch "Sketch1 (2)" against normal blind 38.1 from surface at -387.35 separate body contours L1 L5 L6 L12 L13 | L1 L7 L10 L14 L15 | A0 | A1 makes body 73 at (-169.3333, -13.7583, -387.35) makes body 74 at (122.7667, -13.7583, -387.35) in component "Sacrificial Rim"
extrude "Extrude2''''" add sketch "Sketch1 (2)" against normal blind 38.1 from surface at -387.35 separate body contours L0 L1 L13 L14 | L2 L5 L6 L8 | L7 L9 L10 L11 makes body 75 at (-186.2667, -123.825, -387.35) makes body 76 at (25.4, 109.0083, -387.35) makes body 77 at (296.3333, -123.825, -387.35) in component "Sacrificial Rim"
extrude "Extrude3'''" add sketch "Sketch1 (2)" along normal blind 38.1 from surface at 19.05 separate body contours L1 L5 L6 L12 L13 | L1 L7 L10 L14 L15 | A0 | A1 makes body 78 at (-169.3333, -13.7583, 19.05) makes body 79 at (122.7667, -13.7583, 19.05) in component "Sacrificial Rim"
extrude "Extrude4''" add sketch "Sketch1 (2)" along normal blind 38.1 from surface at 19.05 separate body contours L0 L1 L13 L14 | L2 L5 L6 L8 | L7 L9 L10 L11 makes body 80 at (-186.2667, -123.825, 19.05) makes body 81 at (25.4, 109.0083, 19.05) makes body 82 at (296.3333, -123.825, 19.05) in component "Sacrificial Rim"
extrude "Extrude1''''''" add sketch "Sketch1 (2)" along normal blind 38.1 from surface at -368.3 separate body contours A0 | A1 makes body 83 at (106.3566, 41.0376, -342.9) makes body 84 at (-96.8434, 41.0376, -342.9) in component "Pegs Saddle"
extrude "Extrude2'''''" add sketch "Sketch1 (2)" against normal blind 38.1 separate body contours A0 | A1 makes body 85 at (106.3566, 41.0376, -25.4) makes body 86 at (-96.8434, 41.0376, -25.4) in component "Pegs Saddle"
move_body "Move1'''" [suppressed] in component "Sacrificial Rim"
move_body "Move2" [suppressed] in component "Sacrificial Rim"
move_body "Move1''''" [suppressed] in component "Saddle"
move_body "Move2'" [suppressed] in component "Saddle"
move_body "Move3" [suppressed] in component "Saddle"
component "Large Box" placed x (1, 0, 0) y (0, 1, 0) z (0, 0, 1) at (0, 0, 0)
component "Moving Walls" placed x (1, 0, 0) y (0, 1, 0) z (0, 0, 1) at (0, 0, 0)
component "Sacrificial Sides" placed x (1, 0, 0) y (0, 1, 0) z (0, 0, 1) at (0, 0, 0)
component "Pegs" placed x (1, 0, 0) y (0, 1, 0) z (0, 0, 1) at (0, 0, 0)
component "Saddle" placed x (1, 0, 0) y (0, 1, 0) z (0, 0, 1) at (0, 0, 0)
component "Sacrificial Rim" placed x (1, 0, 0) y (0, 1, 0) z (0, 0, 1) at (0, 0, 0)
component "Pegs Saddle" placed x (1, 0, 0) y (0, 1, 0) z (0, 0, 1) at (0, 0, 0)
hidden bodies 1 3 14 26 45 36 35 47 37 25 24 49 18 19 28 17 34 48 27 15 46 16 38
equation "d128 = ( 3 / 8 ) * 1 in"
equation "d131 = d128"
equation "d132 = d129"
equation "d199 = ( 3 / 8 ) * 1 in"
equation "d202 = d128"
equation "d203 = d129"
equation "d264 = ( 3 / 8 ) * 1 in"
equation "d267 = d128"
equation "d268 = d129"
equation "d329 = ( 3 / 8 ) * 1 in"
equation "d340 = d329"
equation "d341 = d330"
